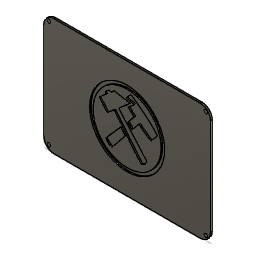
Bandeja Feldherr Tapa Masons (Autodesk Fusion 360 design; units mm, degrees)
Autodesk Fusion 360 part; units mm, degrees
sketch "Base" plane through (0, 0, 0) normal (0, 0, 1) x (1, 0, 0)
  line L0 (0, 0) -> (245, 0)
  line L1 (245, 0) -> (245, -172)
  line L2 (245, -172) -> (0, -172)
  line L3 (0, -172) -> (0, 0)
  circle A0 centre (15, -15) radius 15
  circle A1 centre (230, -15) radius 15
  circle A2 centre (15, -157) radius 15
  circle A3 centre (230, -157) radius 15
  dimension "d4" = 172
  dimension "d5" = 245
  dimension "d6" = 30
  dimension "d7" = 30
  dimension "d8" = 30
  dimension "d9" = 30
  constraint horizontal L0
  constraint vertical L1
  constraint horizontal L2
  constraint vertical L3
  constraint coincident L0.start L3.end
  constraint tangent L0 A0
  constraint tangent L3 A0
  constraint tangent L0 A1
  constraint tangent L1 A1
  constraint tangent L1 A3
  constraint tangent L2 A3
  constraint tangent L2 A2
  constraint tangent L3 A2
  measures "d4" distance of L0.start L2.end
  measures "d5" distance of L0.start L0.end
  measures "d6" diameter of A0
  measures "d7" diameter of A1
  measures "d8" diameter of A2
  measures "d9" diameter of A3
extrude "Extrude1" add sketch "Base" along normal blind 2.5 contours L0 L1 L2 L3 A0 A1 A2 A3 | A0 | A1 | A2 | A3
sketch "Pared" plane through (0, 0, 2.5) normal (0, 0, 1) x (1, 0, 0)
  arc A0 (15, 0) -> (0, -15) centre (15, -15) ccw
  line L0 (0, -15) -> (0, -157)
  arc A1 (0, -157) -> (15, -172) centre (15, -157) ccw
  line L1 (15, -172) -> (230, -172)
  arc A2 (230, -172) -> (245, -157) centre (230, -157) ccw
  line L2 (245, -157) -> (245, -15)
  arc A3 (245, -15) -> (230, 0) centre (230, -15) ccw
  line L3 (230, 0) -> (15, 0)
  line L4 (2, -2) -> (243, -2)
  line L5 (243, -2) -> (243, -170)
  line L6 (243, -170) -> (2, -170)
  line L7 (2, -170) -> (2, -2)
  circle A4 centre (15, -157) radius 13
  circle A5 centre (15, -15) radius 13
  circle A6 centre (230, -15) radius 13
  circle A7 centre (230, -157) radius 13
  line L8 (0, 0) -> (15, -15) construction
  line L9 (4.3934, -4.3934) -> (5.8076, -5.8076) construction
  line L10 (243, -2) -> (230, -15) construction
  line L11 (243, -2) -> (258.3137, -2) construction
  line L12 (240.6066, -4.3934) -> (239.1924, -5.8076) construction
  line L13 (243, -170) -> (230, -157) construction
  line L14 (243, -170) -> (258.3137, -170) construction
  line L15 (240.6066, -167.6066) -> (239.1924, -166.1924) construction
  line L16 (2, -170) -> (15, -157) construction
  line L17 (2, -170) -> (14.3137, -170) construction
  line L18 (4.3934, -167.6066) -> (5.8076, -166.1924) construction
  dimension "d12" = 2
  dimension "d13" = 2
  dimension "d14" = 2
  dimension "d15" = 2
  dimension "d53" = 2
  dimension "d55" = 135
  dimension "d56" = 2
  dimension "d57" = 135
  dimension "d58" = 2
  dimension "d59" = 45
  dimension "d60" = 2
  constraint horizontal L4
  constraint vertical L5
  constraint horizontal L6
  constraint vertical L7
  constraint tangent L7 A4
  constraint tangent L4 A5
  constraint tangent L4 A6
  constraint tangent L5 A7
  constraint tangent L7 A5
  constraint tangent L5 A6
  constraint tangent L6 A7
  constraint tangent L6 A4
  constraint coincident L8.start origin
  constraint coincident A0.centre A5.centre
  constraint coincident A0 L9.start
  constraint coincident A5 L9.end
  constraint collinear L8 L9
  constraint horizontal L11
  constraint coincident A3.centre A6.centre
  constraint coincident A3 L12.start
  constraint coincident A6 L12.end
  constraint collinear L10 L12
  constraint horizontal L14
  constraint coincident A2.centre A7.centre
  constraint coincident A2 L15.start
  constraint coincident A7 L15.end
  constraint collinear L13 L15
  constraint horizontal L17
  constraint coincident A1.centre A4.centre
  constraint coincident A1 L18.start
  constraint coincident A4 L18.end
  constraint collinear L16 L18
  measures "d12" distance of L3 L4
  measures "d13" distance of L0 L7
  measures "d14" distance of L1 L6
  measures "d15" distance of L2 L5
  measures "d53" distance of L9.start L9.end
  measures "d55" angle of L10 L11
  measures "d56" distance of L12.start L12.end
  measures "d57" angle of L13 L14
  measures "d58" distance of L15.start L15.end
  measures "d59" angle of L16 L17
  measures "d60" distance of L18.start L18.end
sketch "Imanes" plane through (0, 0, 0) normal (0, 0, -1) x (-1, 0, 0)
  circle A0 centre (-7.2218, -7.2218) radius 4
  circle A1 centre (-15, -15) radius 15 construction
  line L0 (0, 0) -> (-15, -15) construction
  circle A2 centre (-7.2218, -7.2218) radius 2.6
  circle A3 centre (-7.2218, -164.7782) radius 4
  circle A4 centre (-237.7782, -164.7782) radius 4
  circle A5 centre (-237.7782, -7.2218) radius 4
  circle A6 centre (-230, -15) radius 15 construction
  circle A7 centre (-230, -157) radius 15 construction
  circle A8 centre (-15, -157) radius 15 construction
  line L1 (0, -172) -> (-15, -157) construction
  line L2 (-245, -172) -> (-230, -157) construction
  line L3 (-245, 0) -> (-230, -15) construction
  circle A9 centre (-237.7782, -7.2218) radius 2.6
  circle A10 centre (-237.7782, -164.7782) radius 2.6
  circle A11 centre (-7.2218, -164.7782) radius 2.6
  point P0 (0, -172)
  point P1 (-245, -172)
  point P2 (-245, 0)
  dimension "d32" = 8
  dimension "d33" = 5.2
  dimension "d43" = 8
  dimension "d44" = 8
  dimension "d45" = 8
  dimension "d46" = 5.2
  dimension "d47" = 5.2
  dimension "d48" = 5.2
  constraint tangent A0 A1
  constraint coincident L0.start origin
  constraint coincident A1.centre L0.end
  constraint concentric A0 A2
  constraint tangent A5 A6
  constraint tangent A3 A8
  constraint coincident P0 L1.start
  constraint coincident A8.centre L1.end
  constraint coincident P1 L2.start
  constraint coincident A7.centre L2.end
  constraint coincident P2 L3.start
  constraint coincident A6.centre L3.end
  constraint coincident A5.centre L3
  constraint concentric A5 A9
  constraint coincident A4.centre L2
  constraint concentric A4 A10
  constraint coincident A0.centre L0
  constraint concentric A3 A11
  constraint coincident L1 A3.centre
  constraint tangent A4 A7
  measures "d32" diameter of A0
  measures "d33" diameter of A2
  measures "d43" diameter of A3
  measures "d44" diameter of A4
  measures "d45" diameter of A5
  measures "d46" diameter of A9
  measures "d47" diameter of A10
  measures "d48" diameter of A11
extrude "Extrude6" cut sketch "Imanes" against normal blind 2 contours A2 | A9 | A10 | A11
sketch "Sketch6" plane through (0, 0, 2.5) normal (0, 0, 1) x (1, 0, 0)
  arc A0 (15, 0) -> (0, -15) centre (15, -15) ccw
  line L0 (0, -15) -> (0, -157)
  arc A1 (0, -157) -> (15, -172) centre (15, -157) ccw
  line L1 (15, -172) -> (230, -172)
  arc A2 (230, -172) -> (245, -157) centre (230, -157) ccw
  line L2 (245, -157) -> (245, -15)
  arc A3 (245, -15) -> (230, 0) centre (230, -15) ccw
  line L3 (230, 0) -> (15, 0)
  circle A4 centre (122.5, -86) radius 50
  line L4 (0, -86) -> (245, -86) construction
  line L5 (122.5, 0) -> (122.5, -172) construction
  line L6 (72.5, -36) -> (172.5, -36) construction
  line L7 (172.5, -36) -> (172.5, -136) construction
  line L8 (172.5, -136) -> (72.5, -136) construction
  line L9 (72.5, -136) -> (72.5, -36) construction
  spline S0 degree 3 poles (97.505, -120.2136) (95.2688, -119.1942) (93.4536, -117.5715) (92.2477, -115.5138) knots 0 0 0 0 1 1 1 1
  spline S1 degree 3 poles (92.2477, -115.5138) (91.3611, -114.0009) (91.2937, -113.6586) (91.7538, -113.0061) knots 0 0 0 0 1 1 1 1
  spline S2 degree 3 poles (91.7538, -113.0061) (92.3098, -112.2178) (108.1378, -94.2351) (111.3615, -90.7292) knots 0 0 0 0 1 1 1 1
  line L10 (111.3615, -90.7292) -> (113.2125, -88.7161)
  line L11 (113.2125, -88.7161) -> (116.4697, -92.7381)
  line L12 (116.4697, -92.7381) -> (119.7269, -96.7602)
  line L13 (119.7269, -96.7602) -> (110.0841, -108.8617)
  spline S3 degree 3 poles (110.0841, -108.8617) (104.3312, -116.0816) (100.173, -120.9596) (99.776, -120.9544) knots 0 0 0 0 1 1 1 1
  spline S4 degree 3 poles (99.776, -120.9544) (99.4101, -120.9498) (98.3881, -120.6162) (97.505, -120.2136) knots 0 0 0 0 1 1 1 1
  spline S5 degree 3 poles (124.2859, -98.176) (114.2885, -85.6509) (105.4374, -74.6409) (104.6168, -73.7093) knots 0 0 0 0 1 1 1 1
  line L14 (104.6168, -73.7093) -> (103.1248, -72.0155)
  line L15 (103.1248, -72.0155) -> (98.1581, -76.2356)
  spline S6 degree 3 poles (98.1581, -76.2356) (95.4264, -78.5567) (93.1449, -80.4027) (93.0881, -80.3379) knots 0 0 0 0 1 1 1 1
  spline S7 degree 3 poles (93.0881, -80.3379) (90.4564, -77.3364) (81.6493, -66.5707) (81.6493, -66.3553) knots 0 0 0 0 1 1 1 1
  spline S8 degree 3 poles (81.6493, -66.3553) (81.6493, -66.132) (87.89, -60.7479) (91.2564, -58.0669) knots 0 0 0 0 1 1 1 1
  spline S9 degree 3 poles (91.2564, -58.0669) (91.3521, -57.9907) (91.2166, -57.7146) (90.9554, -57.4534) knots 0 0 0 0 1 1 1 1
  spline S10 degree 3 poles (90.9554, -57.4534) (90.2829, -56.7809) (90.3666, -55.0715) (91.1251, -53.9886) knots 0 0 0 0 1 1 1 1
  spline S11 degree 3 poles (91.1251, -53.9886) (92.116, -52.5738) (94.8993, -50.7164) (96.0284, -50.7164) knots 0 0 0 0 1 1 1 1
  spline S12 degree 3 poles (96.0284, -50.7164) (96.585, -50.7164) (97.3612, -51.0067) (97.7533, -51.3616) knots 0 0 0 0 1 1 1 1
  spline S13 degree 3 poles (97.7533, -51.3616) (98.4178, -51.9629) (98.6422, -51.8575) (101.0546, -49.8109) knots 0 0 0 0 1 1 1 1
  line L16 (101.0546, -49.8109) -> (103.6429, -47.6151)
  line L17 (103.6429, -47.6151) -> (115.1682, -49.7441)
  spline S14 degree 3 poles (115.1682, -49.7441) (121.5071, -50.915) (126.7513, -51.9309) (126.822, -52.0015) knots 0 0 0 0 1 1 1 1
  spline S15 degree 3 poles (126.822, -52.0015) (126.8927, -52.0722) (123.1778, -55.2833) (118.5667, -59.1372) knots 0 0 0 0 1 1 1 1
  spline S16 degree 3 poles (118.5667, -59.1372) (111.3647, -65.1566) (110.255, -66.2311) (110.6944, -66.7597) knots 0 0 0 0 1 1 1 1
  spline S17 degree 3 poles (110.6944, -66.7597) (113.0534, -69.5972) (123.2463, -81.2864) (130.8317, -89.853) knots 0 0 0 0 1 1 1 1
  spline S18 degree 3 poles (130.8317, -89.853) (152.1798, -113.9625) (151.5983, -113.2705) (151.3475, -114.2699) knots 0 0 0 0 1 1 1 1
  spline S19 degree 3 poles (151.3475, -114.2699) (150.8986, -116.0584) (148.366, -118.8432) (146.2122, -119.9165) knots 0 0 0 0 1 1 1 1
  spline S20 degree 3 poles (146.2122, -119.9165) (145.0569, -120.4922) (143.7408, -120.96) (143.2874, -120.9561) knots 0 0 0 0 1 1 1 1
  spline S21 degree 3 poles (143.2874, -120.9561) (142.6826, -120.9504) (137.6207, -114.8823) (124.2859, -98.176) knots 0 0 0 0 1 1 1 1
  spline S22 degree 3 poles (150.8471, -80.2857) (147.2897, -77.821) (143.3323, -74.9401) (142.0529, -73.8835) knots 0 0 0 0 1 1 1 1
  line L18 (142.0529, -73.8835) -> (139.7267, -71.9624)
  line L19 (139.7267, -71.9624) -> (138.4857, -73.4534)
  spline S23 degree 3 poles (138.4857, -73.4534) (137.8031, -74.2734) (135.5505, -77.0345) (133.4798, -79.5892) knots 0 0 0 0 1 1 1 1
  spline S24 degree 3 poles (133.4798, -79.5892) (131.4091, -82.1439) (129.6028, -84.1445) (129.4657, -84.0349) knots 0 0 0 0 1 1 1 1
  spline S25 degree 3 poles (129.4657, -84.0349) (129.3286, -83.9253) (127.881, -82.3387) (126.2488, -80.5091) knots 0 0 0 0 1 1 1 1
  line L20 (126.2488, -80.5091) -> (123.2812, -77.1827)
  line L21 (123.2812, -77.1827) -> (124.0838, -76.2929)
  spline S26 degree 3 poles (124.0838, -76.2929) (124.5252, -75.8035) (126.6439, -73.3539) (128.7921, -70.8493) knots 0 0 0 0 1 1 1 1
  line L22 (128.7921, -70.8493) -> (132.6978, -66.2954)
  line L23 (132.6978, -66.2954) -> (128.3816, -62.2081)
  line L24 (128.3816, -62.2081) -> (124.0654, -58.1208)
  line L25 (124.0654, -58.1208) -> (128.5839, -54.3545)
  spline S27 degree 3 poles (128.5839, -54.3545) (131.6844, -51.7701) (132.9335, -50.4982) (132.5643, -50.3014) knots 0 0 0 0 1 1 1 1
  spline S28 degree 3 poles (132.5643, -50.3014) (132.2684, -50.1437) (129.6781, -49.6074) (126.808, -49.1095) knots 0 0 0 0 1 1 1 1
  spline S29 degree 3 poles (126.808, -49.1095) (123.9379, -48.6117) (121.45, -48.1241) (121.2793, -48.026) knots 0 0 0 0 1 1 1 1
  spline S30 degree 3 poles (121.2793, -48.026) (121.1086, -47.9279) (122.4543, -46.0997) (124.2697, -43.9633) knots 0 0 0 0 1 1 1 1
  spline S31 degree 3 poles (124.2697, -43.9633) (126.0852, -41.827) (127.6096, -40.0189) (127.6573, -39.9455) knots 0 0 0 0 1 1 1 1
  spline S32 degree 3 poles (127.6573, -39.9455) (127.9102, -39.5561) (141.6791, -49.53) (146.8741, -53.8656) knots 0 0 0 0 1 1 1 1
  spline S33 degree 3 poles (146.8741, -53.8656) (156.1212, -61.5832) (157.8959, -63.2062) (162.6831, -68.3239) knots 0 0 0 0 1 1 1 1
  line L26 (162.6831, -68.3239) -> (167.1242, -73.0715)
  line L27 (167.1242, -73.0715) -> (162.2715, -78.8535)
  spline S34 degree 3 poles (162.2715, -78.8535) (159.6025, -82.0337) (157.3955, -84.6651) (157.367, -84.7012) knots 0 0 0 0 1 1 1 1
  spline S35 degree 3 poles (157.367, -84.7012) (157.3385, -84.7373) (154.4045, -82.7503) (150.8471, -80.2857) knots 0 0 0 0 1 1 1 1
  circle A5 centre (122.5, -86) radius 55
  line L28 (172.5, -136) -> (72.5, -36) construction
  line L29 (172.5, -36) -> (72.5, -136) construction
  dimension "d73" = 100
  dimension "d74" = 110
  constraint midpoint L0 L4.start
  constraint midpoint L2 L4.end
  constraint midpoint L3 L5.start
  constraint midpoint L1 L5.end
  constraint coincident A4.centre L4
  constraint coincident A4.centre L5
  constraint horizontal L6
  constraint vertical L7
  constraint horizontal L8
  constraint vertical L9
  constraint tangent A4 L6
  constraint tangent A4 L9
  constraint tangent A4 L8
  constraint tangent A4 L7
  constraint concentric A4 A5
  measures "d73" diameter of A4
  measures "d74" diameter of A5
extrude "Extrude8" cut sketch "Sketch6" against normal blind 2 contours S0 S1 S2 L10 L11 L12 L13 S3 S4 | S5 L14 L15 S6 S7 S8 S9 S10 S11 S12 S13 L16 L17 S14 S15 S16 S17 S18 S19 S20 S21 | S22 L18 L19 S23 S24 S25 L20 L21 S26 L22 L23 L24 L25 S27 S28 S29 S30 S31 S32 S33 L26 L27 S34 S35 | A5
equation "d4 = bandeja_y"
equation "d5 = bandeja_x"
equation "d6 = bandeja_filet"
equation "d7 = bandeja_filet"
equation "d8 = bandeja_filet"
equation "d9 = bandeja_filet"
equation "d10 = extrusion_bandeja_piso"
equation "d12 = bandeja_pared"
equation "d13 = bandeja_pared"
equation "d14 = bandeja_pared"
equation "d15 = bandeja_pared"
equation "d32 = iman_pared"
equation "d33 = iman_diametro"
equation "d37 = -extrusion_iman_inferior"
equation "d43 = iman_pared"
equation "d44 = iman_pared"
equation "d45 = iman_pared"
equation "d46 = iman_diametro"
equation "d47 = iman_diametro"
equation "d48 = iman_diametro"
equation "d53 = bandeja_pared"
equation "d56 = bandeja_pared"
equation "d58 = bandeja_pared"
equation "d60 = bandeja_pared"
equation "bandeja_x = 245 mm"
equation "bandeja_y = 172 mm"
equation "bandeja_filet = 30 mm"
equation "bandeja_pared = 2 mm"
equation "iman_diametro = 5.2 mm"
equation "iman_pared = iman_diametro + 2.8 mm"
equation "extrusion_bandeja_piso = 2.5 mm"
equation "extrusion_iman_inferior = 2 mm"
equation "d75 = -extrusion_logo"
equation "extrusion_logo = 2 mm"
named bodies: "Bandeja Feldherr Tapa Masons"
